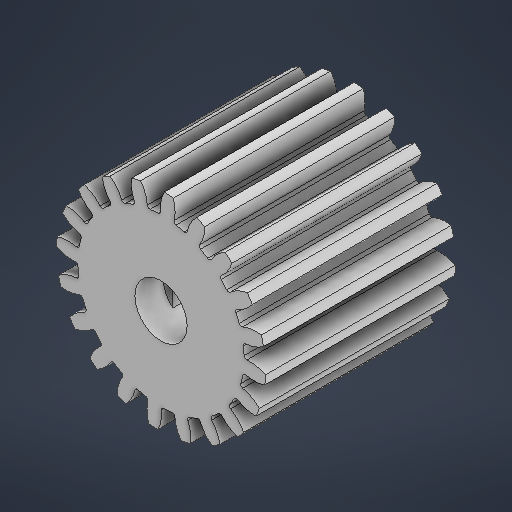
# Autodesk Inventor part: piñon 4
Saved by Autodesk Inventor 2025.3 (Build 293356000, 356)
## iProperties
Created: 2025-10-14
Part Number: piñon 4
Material: Genérico
Document SubType Name: Modeling
Designer: Jonathan Galarza
Density: 1 g/cm^3
Appearance: Valor por defecto
Author: Jonathan Galarza
Autodesk Inventor part; units mm, degrees
ref_plane "YZ Plane" through (0, 0, 0) normal (1, 0, 0) x (0, 1, 0)
ref_plane "XZ Plane" through (0, 0, 0) normal (0, 1, 0) x (-1, 0, 0)
ref_plane "XY Plane" through (0, 0, 0) normal (0, 0, 1) x (1, 0, 0)
sketch "Boceto1" plane through (0, 0, 0) normal (0, 0, 1) x (1, 0, 0)
  arc A0 (10.9229, -1.2998) -> (10.9948, -0.3367) centre (0, 0) ccw
  circle A1 centre (0, 0) radius 8.75
  line L0 (0, 0) -> (10, 0) construction
  line L1 (0, 0) -> (10, 0) construction
  line L2 (0, 0) -> (9.8891, -1.485) construction
  line L3 (0, 0) -> (10, 0) construction
  arc A2 (10.9948, -0.3367) -> (8.75, -0.008) centre (9.3969, -3.4202) ccw
  arc A3 (8.6542, -1.2914) -> (10.9229, -1.2998) centre (9.8006, 1.9868) ccw
  arc A4 (10.5608, 3.0774) -> (8.3242, 2.6963) centre (9.9939, -0.349) ccw
  arc A5 (10.79, 2.1392) -> (10.5608, 3.0774) centre (0, 0) ccw
  arc A6 (8.6297, 1.4461) -> (10.79, 2.1392) centre (8.707, 4.9182) ccw
  arc A7 (9.0929, 6.1902) -> (7.0836, 5.1366) centre (9.6126, 2.7564) ccw
  arc A8 (9.6008, 5.3688) -> (9.0929, 6.1902) centre (0, 0) ccw
  arc A9 (7.7605, 4.042) -> (9.6008, 5.3688) centre (6.761, 7.3681) ccw
  arc A10 (6.735, 8.6971) -> (5.1496, 7.0742) centre (8.2904, 5.5919) ccw
  arc A11 (7.4719, 8.0728) -> (6.735, 8.6971) centre (0, 0) ccw
  arc A12 (6.1316, 6.2423) -> (7.4719, 8.0728) centre (4.1533, 9.0967) ccw
  arc A13 (3.7178, 10.3527) -> (2.7115, 8.3193) centre (6.1566, 7.8801) ccw
  arc A14 (4.6115, 9.9867) -> (3.7178, 10.3527) centre (0, 0) ccw
  arc A15 (3.9025, 7.8315) -> (4.6115, 9.9867) centre (1.139, 9.9349) ccw
  arc A16 (0.3367, 10.9948) -> (0.008, 8.75) centre (3.4202, 9.3969) ccw
  arc A17 (1.2998, 10.9229) -> (0.3367, 10.9948) centre (0, 0) ccw
  arc A18 (1.2914, 8.6542) -> (1.2998, 10.9229) centre (-1.9868, 9.8006) ccw
  arc A19 (-3.0774, 10.5608) -> (-2.6963, 8.3242) centre (0.349, 9.9939) ccw
  arc A20 (-2.1392, 10.79) -> (-3.0774, 10.5608) centre (0, 0) ccw
  arc A21 (-1.4461, 8.6297) -> (-2.1392, 10.79) centre (-4.9182, 8.707) ccw
  arc A22 (-6.1902, 9.0929) -> (-5.1366, 7.0836) centre (-2.7564, 9.6126) ccw
  arc A23 (-5.3688, 9.6008) -> (-6.1902, 9.0929) centre (0, 0) ccw
  arc A24 (-4.042, 7.7605) -> (-5.3688, 9.6008) centre (-7.3681, 6.761) ccw
  arc A25 (-8.6971, 6.735) -> (-7.0742, 5.1496) centre (-5.5919, 8.2904) ccw
  arc A26 (-8.0728, 7.4719) -> (-8.6971, 6.735) centre (0, 0) ccw
  arc A27 (-6.2423, 6.1316) -> (-8.0728, 7.4719) centre (-9.0967, 4.1533) ccw
  arc A28 (-10.3527, 3.7178) -> (-8.3193, 2.7115) centre (-7.8801, 6.1566) ccw
  arc A29 (-9.9867, 4.6115) -> (-10.3527, 3.7178) centre (0, 0) ccw
  arc A30 (-7.8315, 3.9025) -> (-9.9867, 4.6115) centre (-9.9349, 1.139) ccw
  arc A31 (-10.9948, 0.3367) -> (-8.75, 0.008) centre (-9.3969, 3.4202) ccw
  arc A32 (-10.9229, 1.2998) -> (-10.9948, 0.3367) centre (0, 0) ccw
  arc A33 (-8.6542, 1.2914) -> (-10.9229, 1.2998) centre (-9.8006, -1.9868) ccw
  arc A34 (-10.5608, -3.0774) -> (-8.3242, -2.6963) centre (-9.9939, 0.349) ccw
  arc A35 (-10.79, -2.1392) -> (-10.5608, -3.0774) centre (0, 0) ccw
  arc A36 (-8.6297, -1.4461) -> (-10.79, -2.1392) centre (-8.707, -4.9182) ccw
  arc A37 (-9.0929, -6.1902) -> (-7.0836, -5.1366) centre (-9.6126, -2.7564) ccw
  arc A38 (-9.6008, -5.3688) -> (-9.0929, -6.1902) centre (0, 0) ccw
  arc A39 (-7.7605, -4.042) -> (-9.6008, -5.3688) centre (-6.761, -7.3681) ccw
  arc A40 (-6.735, -8.6971) -> (-5.1496, -7.0742) centre (-8.2904, -5.5919) ccw
  arc A41 (-7.4719, -8.0728) -> (-6.735, -8.6971) centre (0, 0) ccw
  arc A42 (-6.1316, -6.2423) -> (-7.4719, -8.0728) centre (-4.1533, -9.0967) ccw
  arc A43 (-3.7178, -10.3527) -> (-2.7115, -8.3193) centre (-6.1566, -7.8801) ccw
  arc A44 (-4.6115, -9.9867) -> (-3.7178, -10.3527) centre (0, 0) ccw
  arc A45 (-3.9025, -7.8315) -> (-4.6115, -9.9867) centre (-1.139, -9.9349) ccw
  arc A46 (-0.3367, -10.9948) -> (-0.008, -8.75) centre (-3.4202, -9.3969) ccw
  arc A47 (-1.2998, -10.9229) -> (-0.3367, -10.9948) centre (0, 0) ccw
  arc A48 (-1.2914, -8.6542) -> (-1.2998, -10.9229) centre (1.9868, -9.8006) ccw
  arc A49 (3.0774, -10.5608) -> (2.6963, -8.3242) centre (-0.349, -9.9939) ccw
  arc A50 (2.1392, -10.79) -> (3.0774, -10.5608) centre (0, 0) ccw
  arc A51 (1.4461, -8.6297) -> (2.1392, -10.79) centre (4.9182, -8.707) ccw
  arc A52 (6.1902, -9.0929) -> (5.1366, -7.0836) centre (2.7564, -9.6126) ccw
  arc A53 (5.3688, -9.6008) -> (6.1902, -9.0929) centre (0, 0) ccw
  arc A54 (4.042, -7.7605) -> (5.3688, -9.6008) centre (7.3681, -6.761) ccw
  arc A55 (8.6971, -6.735) -> (7.0742, -5.1496) centre (5.5919, -8.2904) ccw
  arc A56 (8.0728, -7.4719) -> (8.6971, -6.735) centre (0, 0) ccw
  arc A57 (6.2423, -6.1316) -> (8.0728, -7.4719) centre (9.0967, -4.1533) ccw
  arc A58 (10.3527, -3.7178) -> (8.3193, -2.7115) centre (7.8801, -6.1566) ccw
  arc A59 (9.9867, -4.6115) -> (10.3527, -3.7178) centre (0, 0) ccw
  arc A60 (7.8315, -3.9025) -> (9.9867, -4.6115) centre (9.9349, -1.139) ccw
  point P0 (9.5106, 3.0902)
  point P1 (8.0902, 5.8779)
  point P2 (5.8779, 8.0902)
  point P3 (3.0902, 9.5106)
  point P4 (0, 10)
  point P5 (-3.0902, 9.5106)
  point P6 (-5.8779, 8.0902)
  point P7 (-8.0902, 5.8779)
  point P8 (-9.5106, 3.0902)
  point P9 (-10, 0)
  point P10 (-9.5106, -3.0902)
  point P11 (-8.0902, -5.8779)
  point P12 (-5.8779, -8.0902)
  point P13 (-3.0902, -9.5106)
  point P14 (0, -10)
  point P15 (3.0902, -9.5106)
  point P16 (5.8779, -8.0902)
  point P17 (8.0902, -5.8779)
  point P18 (9.5106, -3.0902)
  point P19 (0.008, 8.75)
  point P20 (-1.4461, 8.6297)
  point P21 (-2.6963, 8.3242)
  point P22 (-5.1366, 7.0836)
  point P23 (-6.2423, 6.1316)
  point P24 (-7.0742, 5.1496)
  point P25 (-8.3193, 2.7115)
  point P26 (-8.6542, 1.2914)
  point P27 (-8.75, 0.008)
  point P28 (-8.6297, -1.4461)
  point P29 (-8.3242, -2.6963)
  point P30 (-7.0836, -5.1366)
  point P31 (-6.1316, -6.2423)
  point P32 (-5.1496, -7.0742)
  point P33 (-3.9025, -7.8315)
  point P34 (-2.7115, -8.3193)
  point P35 (-1.2914, -8.6542)
  point P36 (-0.008, -8.75)
  point P37 (5.1366, -7.0836)
  point P38 (6.2423, -6.1316)
  point P39 (7.8315, -3.9025)
  point P40 (8.3193, -2.7115)
  point P41 (8.6542, -1.2914)
  point P42 (8.6297, 1.4461)
  point P43 (8.3242, 2.6963)
  point P44 (7.0836, 5.1366)
  point P45 (6.1316, 6.2423)
  point P46 (5.1496, 7.0742)
  point P47 (2.7115, 8.3193)
  point P48 (1.2914, 8.6542)
  point P49 (2.6963, -8.3242)
  point P50 (1.4461, -8.6297)
  dimension "d6" = 8.54
  dimension "d9" = 360
  constraints: 140 point on circle, 60 centre point, 8 end point, 3 coincident, 3 horizontal, 1 equal length, 225 other
  measures "d6" angle of L2 L3
extrude "Extrusión1" add sketch "Boceto1" along normal blind 20
sketch "Boceto2" plane through (0, 0, 20) normal (0, 0, 1) x (1, 0, 0)
  circle A0 centre (0, 0) radius 2.75
  line L0 (-1.75, 0) -> (1.75, 0) construction
  line L1 (-1.75, 2.1213) -> (-1.75, -2.1213)
  line L2 (1.75, 2.1213) -> (1.75, -2.1213)
  dimension "d13" = 5.5
  constraints: 6 end point, 4 point on circle, 3 midpoint, 2 coincident, 2 vertical, 1 centre point, 1 horizontal
  measures "d13" diameter of A0
extrude "Extrusión2" cut sketch "Boceto2" against normal through all contours L2 A0 L1
fillet "Empalme1" radius 0.261 2 edges at (-8.3193, 2.7115, 10) (-7.8315, 3.9025, 10)
pattern_circular "Patrón circular1" count 20 over 360 about axis through (0, 0, 0) along (0, 0, 1) of "Empalme1"
sketch "Boceto3" plane through (0, 0, 0) normal (0, 0, -1) x (-1, 0, 0)
  arc A0 (1.75, 2.1213) -> (-1.75, 2.1213) centre (0, 0) ccw construction
  arc A1 (1.75, 2.1213) -> (-1.75, 2.1213) centre (0, 0) ccw construction
  arc A2 (-1.75, -2.1213) -> (1.75, -2.1213) centre (0, 0) ccw projected
  arc A3 (-1.75, -2.1213) -> (1.75, -2.1213) centre (0, 0) ccw projected
  circle A4 centre (0, 0) radius 2.75
  point P0 (1.3748, -8.9284)
  point P1 (1.75, -2.1213)
  dimension "d22" = 5.5
  constraints: 1 centre point, 1 coincident
  measures "d22" diameter of A4
extrude "Extrusión3" cut sketch "Boceto3" against normal blind 5
sketch "Boceto4" plane through (0, 0, 20) normal (0, 0, 1) x (1, 0, 0)
  circle A0 centre (0, 0) radius 2.75
  dimension "d25" = 5.5
  constraints: 1 centre point, 1 coincident
  measures "d25" diameter of A0
extrude "Extrusión4" cut sketch "Boceto4" against normal blind 3
